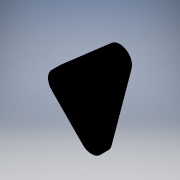
# Autodesk Inventor part: アーム抑えツイン1
Saved by Autodesk Inventor 2020 (Build 240168000, 168)
## iProperties
Created: 2018-12-10
Part Number: アーム抑えツイン1
Material: ポリカーボネート、クリア
Document SubType Name: Modeling
Designer: 雪村
Density: 1.2 g/cm^3
Appearance: 陽極酸化 - 黒
Mass: 2.03192 g
Surface Area: 15.0999 cm^2
Volume: 1.69327 cm^3
Description: ポリカ 3t
Author: 雪村
Autodesk Inventor part; units mm, degrees
ref_plane "YZ Plane" through (0, 0, 0) normal (1, 0, 0) x (0, 1, 0)
ref_plane "XZ Plane" through (0, 0, 0) normal (0, 1, 0) x (-1, 0, 0)
ref_plane "XY Plane" through (0, 0, 0) normal (0, 0, 1) x (1, 0, 0)
sketch "スケッチ1" plane through (0, 0, 0) normal (0, 0, 1) x (1, 0, 0)
  circle A0 centre (-165.8946, -3.3102) radius 1.5
  circle A1 centre (-136.5368, 15.7454) radius 1.5
  circle A2 centre (-82.4879, 34.801) radius 1.5
  circle A3 centre (-77.8211, 53.8566) radius 1.5
  circle A4 centre (-107.1789, 34.801) radius 1.5
  circle A5 centre (-110.4783, 13.7882) radius 1.5
  circle A6 centre (-138.4687, -7.2246) radius 1.5
  circle A7 centre (-184.7359, -19.7422) radius 1.5
  circle A8 centre (-173.2477, -31.458) radius 1.5
  circle A9 centre (-44.4492, 64.0137) radius 1.5
  circle A10 centre (-64.4423, 49.0046) radius 1.5
  circle A11 centre (-60.4494, 64.5064) radius 1.5
  line L0 (-64.2741, 70.3989) -> (-190.1939, -11.3332)
  arc A12 (-190.1939, -11.3332) -> (-190.9729, -27.5907) centre (-184.7359, -19.7422) ccw
  line L1 (-190.9729, -27.5907) -> (-178.2249, -37.7212)
  arc A13 (-178.2249, -37.7212) -> (-168.4448, -37.8558) centre (-173.2477, -31.458) ccw
  line L2 (-168.4448, -37.8558) -> (-40.2316, 58.3956)
  arc A14 (-40.2316, 58.3956) -> (-44.233, 71.0354) centre (-44.4492, 64.0137) ccw
  line L3 (-44.233, 71.0354) -> (-60.2332, 71.5281)
  arc A15 (-60.2332, 71.5281) -> (-64.2741, 70.3989) centre (-60.4494, 64.5064) ccw
  arc A16 (-161.5407, -4.4476) -> (-168.8524, 0.0812) centre (-165.8946, -3.3102) ccw
  arc A17 (-187.6936, -16.3507) -> (-187.9489, -22.8928) centre (-184.7359, -19.7422) ccw
  arc A18 (-176.4608, -34.6086) -> (-168.8938, -32.5954) centre (-173.2477, -31.458) ccw
  line L4 (-187.6936, -16.3507) -> (-168.8524, 0.0812)
  line L5 (-161.5407, -4.4476) -> (-168.8938, -32.5954)
  line L6 (-187.9489, -22.8928) -> (-176.4608, -34.6086)
  point P0 (0, 0)
  point P1 (0, 0)
  dimension "d0" = 3
  dimension "d1" = 3
  dimension "d2" = 3
  constraints: 19 centre point, 14 end point, 14 point on circle, 6 tangent, 46 other
  measures "d0" radial gap between concentric circles of A0 A16
  measures "d1" radial gap between concentric circles of A7 A17
  measures "d2" radial gap between concentric circles of A8 A18
extrude "押し出し1" add sketch "スケッチ1" along normal blind 3 contours L5 A18 L6 A17 L4 A16
